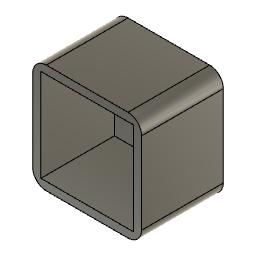
_Caixinha Morea.412478a3-86b5-4890-a604-105011969214 - Copia (Autodesk Fusion 360 design; units mm, degrees)
Autodesk Fusion 360 part; units mm, degrees
box "BoxPrimitive1" add length 200 width 200 height 150 placed x (0, 0, 1) y (1, 0, 0) z (0, 1, 0) at (0, 0, 0) makes body 1
shell "Shell1" thickness 15 removed faces 1 at (133.3333, 0, 66.6667) on bodies 1
fillet "Fillet1" radius 25 1 edges at (0, 75, 200) on bodies 1
fillet "Fillet2" radius 25 3 edges at (200, 75, 200) (0, 75, 0) (200, 75, 0) on bodies 1
cylinder "CylinderPrimitive1" add diameter 40 height 200 placed x (1, 0, 0) y (0, 0, -1) z (0, 1, 0) at (-160, 0, 30) separate body makes body 2
delete_face "DeleteFace1" 3 faces at (-155.2577, 0, 37.1112) (-140.0994, 66.6667, 28.0086) (-155.2577, 200, 37.1112) on bodies 2
hole "Hole1" at (97.506, 135, 43.5548) direction (0, 1, 0) diameter 17 depth 80 tip angle 118 bodies 1
